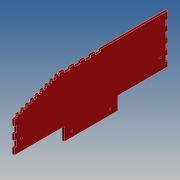
# Autodesk Inventor part: KB33-046-004-007 - Центральная левая боковая пластина
Saved by Autodesk Inventor 2020 (Build 240168000, 168)
## iProperties
Created: 2021-06-25
Part Number: KB33-046-004-007 - Центральная левая боковая пластина
Material: Типовые
Document SubType Name: Modeling
Designer: Петров Иван
Density: 1 g/cm^3
Appearance: По умолчанию
Mass: 113.587 g
Surface Area: 610.329 cm^2
Volume: 113.587 cm^3
Author: Петров Иван
Autodesk Inventor part; units mm, degrees
ref_plane "YZ Plane" through (0, 0, 0) normal (1, 0, 0) x (0, 1, 0)
ref_plane "XZ Plane" through (0, 0, 0) normal (0, 1, 0) x (-1, 0, 0)
ref_plane "XY Plane" through (0, 0, 0) normal (0, 0, 1) x (1, 0, 0)
sketch "Эскиз1" plane through (0, 0, 0) normal (1, 0, 0) x (0, 1, 0)
  line L0 (-10.528, 98.8876) -> (15, 98.8876)
  line L1 (15, 98.8876) -> (15, -5.1124)
  line L2 (15, -5.1124) -> (-10.528, -5.1124)
  line L3 (-10.528, -5.1124) -> (-10.528, 98.8876)
  point P0 (0, 0)
  dimension "d0" = 25.528
  dimension "d1" = 104
  constraints: 8 end point, 2 parallel, 1 horizontal, 1 perpendicular
  measures "d0" distance of L1.end L2.end
  measures "d1" distance of L0.end L1.end
extrude "Выдавливание1" add sketch "Эскиз1" along normal blind 4
sketch "Эскиз2" plane through (4, 0, 0) normal (1, 0, 0) x (0, 0, -1)
  circle A0 centre (-9.8876, -0.528) radius 2 projected
  circle A1 centre (-83.8876, -0.528) radius 2 projected
  point P0 (0, 0)
extrude "Выдавливание2" cut sketch "Эскиз2" against normal blind 4
sketch "Эскиз3" plane through (4, 0, 0) normal (1, 0, 0) x (0, 0, -1)
  line L0 (-191.6906, 75) -> (97.9154, 75)
  line L1 (97.9154, 75) -> (97.9154, 15)
  line L2 (97.9154, 15) -> (-191.6906, 15)
  line L3 (-191.6906, 15) -> (-191.6906, 75)
  line L4 (-98.8876, 15) -> (-98.8876, -10.528) projected
  line L5 (5.1124, -10.528) -> (5.1124, 15) projected
  point P0 (0, 0)
  dimension "d6" = 92.803
  dimension "d7" = 92.803
  dimension "d8" = 60
  constraints: 8 end point, 2 parallel, 1 horizontal, 1 perpendicular, 1 point on line
  measures "d6" distance between parallel lines of L3 L4
  measures "d7" distance between parallel lines of L1 L5
  measures "d8" distance between parallel lines of L2 L0
extrude "Выдавливание3" add sketch "Эскиз3" against normal blind 4
sketch "Эскиз4" plane through (4, 0, 0) normal (1, 0, 0) x (0, 0, -1)
  line L0 (-191.6906, 75) -> (97.9154, 75) projected
  line L1 (-191.6906, 75) -> (-109.2663, 105)
  line L2 (-109.2663, 105) -> (97.9154, 105)
  line L3 (97.9154, 105) -> (97.9154, 75)
  line L4 (97.9154, 75) -> (-191.6906, 75) projected
  line L5 (-98.8876, -10.528) -> (5.1124, -10.528) projected
  line L6 (-46.8876, -10.528) -> (-46.8876, 5.327)
  point P0 (0, 0)
  dimension "d11" = 30
  dimension "d12" = 90
  dimension "d15" = 20
  constraints: 8 end point, 1 midpoint, 1 parallel, 1 vertical
  measures "d11" distance between parallel lines of L0 L2
  measures "d12" angle of L0 L3
  measures "d15" angle of L0 L1
extrude "Выдавливание4" add sketch "Эскиз4" against normal blind 4
sketch "Эскиз5" plane through (0, 15, 191.6906) normal (0, 0, 1) x (1, 0, 0)
  line L0 (0, 0) -> (0, 60) projected
  line L1 (4, 60) -> (4, 0) projected
  line L2 (0, 60) -> (4, 60)
  line L3 (4, 60) -> (4, 48)
  line L4 (4, 48) -> (0, 48)
  line L5 (0, 48) -> (0, 60)
  point P0 (0, -15)
  point P1 (0, 48)
  dimension "d16" = 12
  constraints: 8 end point, 2 parallel, 1 horizontal, 1 perpendicular, 1 point on line
  measures "d16" distance of L2.end L3.end
extrude "Выдавливание5" add sketch "Эскиз5" along normal blind 4
pattern_linear "Прямоуг.массив1" count 3 spacing 24 along (0, -1, 0) of "Выдавливание5"
sketch "Эскиз6" plane through (4, 15, -97.9154) normal (0, 0, -1) x (-1, 0, 0)
  line L0 (4, 90) -> (4, 0) projected
  line L1 (0, 90) -> (4, 90)
  line L2 (4, 90) -> (4, 80)
  line L3 (4, 80) -> (0, 80)
  line L4 (0, 80) -> (0, 90)
  point P0 (4, -15)
  dimension "d22" = 10
  constraints: 8 end point, 2 parallel, 1 horizontal, 1 perpendicular, 1 point on line
  measures "d22" distance of L1.end L2.end
extrude "Выдавливание6" add sketch "Эскиз6" along normal blind 4
pattern_linear "Прямоуг.массив2" count 5 spacing 20 along (0, -1, 0) of "Выдавливание6"
sketch "Эскиз7" plane through (4, 0, 0) normal (1, 0, 0) x (0, 0, -1)
  line L0 (-109.2663, 105) -> (101.9154, 105) projected
  line L1 (101.9154, 105) -> (91.9154, 105)
  line L2 (91.9154, 105) -> (91.9154, 109)
  line L3 (91.9154, 109) -> (101.9154, 109)
  line L4 (101.9154, 109) -> (101.9154, 105)
  point P0 (0, 0)
  dimension "d28" = 10
  dimension "d29" = 4
  constraints: 8 end point, 2 parallel, 1 horizontal, 1 perpendicular
  measures "d28" distance of L2.end L3.end
  measures "d29" distance of L1.end L2.end
extrude "Выдавливание7" add sketch "Эскиз7" against normal blind 4
pattern_linear "Прямоуг.массив3" count 11 spacing 20 along (0, 0, 1) of "Выдавливание7"
sketch "Эскиз8" plane through (4, 0, 0) normal (1, 0, 0) x (0, 0, -1)
  circle A0 centre (-182.1718, 36.9996) radius 2 projected
  circle A1 centre (88.3965, 36.9996) radius 2 projected
  point P0 (0, 0)
extrude "Выдавливание8" cut sketch "Эскиз8" against normal blind 4
sketch "Эскиз9" plane through (0, 105, 109.2663) normal (0, 0.9396926, 0.3420201) x (1, 0, 0)
  line L0 (4, 0) -> (0, 0) projected
  line L1 (4, -29.7601) -> (4, 67.9679) projected
  line L2 (0, 0) -> (4, 0)
  line L3 (4, 0) -> (4, -5)
  line L4 (4, -5) -> (0, -5)
  line L5 (0, -5) -> (0, 0)
  point P0 (0, 66.7646)
  dimension "d37" = 5
  constraints: 8 end point, 2 parallel, 1 horizontal, 1 perpendicular, 1 point on line
  measures "d37" distance of L2.end L3.end
extrude "Выдавливание9" add sketch "Эскиз9" along normal blind 4
pattern_linear "Прямоуг.массив4" count 9 spacing 10 along (0, -0.3420201, 0.9396926) of "Выдавливание9"
sketch "Эскиз10" plane through (4, 0, 0) normal (1, 0, 0) x (0, 0, -1)
  line L0 (101.9154, 109) -> (91.9154, 109) projected
  line L1 (101.9154, 109) -> (-23.0846, 109)
  line L2 (-23.0846, 109) -> (-23.0846, 105)
  line L3 (-23.0846, 105) -> (101.9154, 105)
  line L4 (101.9154, 105) -> (101.9154, 109)
  point P0 (0, 0)
  dimension "d43" = 125
  constraints: 8 end point, 2 parallel, 1 horizontal, 1 perpendicular
  measures "d43" distance of L3.end L2.end
extrude "Выдавливание10" add sketch "Эскиз10" against normal blind 4
equation "\"d7\" = d6"
